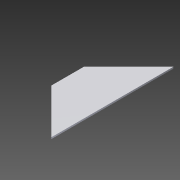
# Autodesk Inventor part: top long
Saved by Autodesk Inventor 2015 (Build 190159000, 159)
## iProperties
Created: 2019-04-10
Part Number: top long
Material: Generic
Document SubType Name: Modeling
Designer: Raptor
Density: 1 g/cm^3
Appearance: Snow
Author: Raptor
Autodesk Inventor part; units mm, degrees
ref_plane "YZ Plane" through (0, 0, 0) normal (1, 0, 0) x (0, 1, 0)
ref_plane "XZ Plane" through (0, 0, 0) normal (0, 1, 0) x (-1, 0, 0)
ref_plane "XY Plane" through (0, 0, 0) normal (0, 0, 1) x (1, 0, 0)
sketch "Sketch4" plane through (0, 0, 0) normal (0, 1, 0) x (-1, 0, 0)
  line L0 (0, 0) -> (0, -1500)
  line L1 (0, -1500) -> (550, -950)
  line L2 (550, -950) -> (550, -550)
  line L3 (550, -550) -> (0, 0)
  dimension "d5" = 45
  dimension "d6" = 45
  dimension "d8" = 1500
  dimension "d11" = 550
  constraints: 8 end point, 1 parallel, 1 vertical
  measures "d5" angle of L3 L0
  measures "d6" angle of L1 L0
  measures "d8" distance of L0.start L0.end
  measures "d11" distance between parallel lines of L0 L2
extrude "Extrusion1" add sketch "Sketch4" along normal blind 20
body "Solid1"
